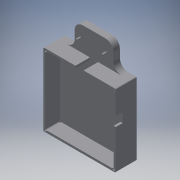
# Autodesk Inventor part: base
Saved by Autodesk Inventor 2019 (Build 230136000, 136)
## iProperties
Created: 2021-10-12
Part Number: base
Material: Generic
Document SubType Name: Modeling
Designer: Pulag
Density: 1 g/cm^3
Appearance: Default
Author: Pulag
Autodesk Inventor part; units mm, degrees
ref_plane "YZ Plane" through (0, 0, 0) normal (1, 0, 0) x (0, 1, 0)
ref_plane "XZ Plane" through (0, 0, 0) normal (0, 1, 0) x (-1, 0, 0)
ref_plane "XY Plane" through (0, 0, 0) normal (0, 0, 1) x (1, 0, 0)
sketch "Sketch1" plane through (0, 0, 0) normal (0, 0, 1) x (1, 0, 0)
  line L0 (-42.25, 42.25) -> (42.25, 42.25)
  line L1 (42.25, 42.25) -> (42.25, -42.25)
  line L2 (42.25, -42.25) -> (-42.25, -42.25)
  line L3 (-42.25, -42.25) -> (-42.25, 42.25)
  line L4 (-42.25, 42.25) -> (42.25, -42.25) construction
  line L5 (42.25, 42.25) -> (-42.25, -42.25) construction
  line L6 (-45, 45) -> (45, 45)
  line L7 (45, 45) -> (45, -45)
  line L8 (45, -45) -> (-45, -45)
  line L9 (-45, -45) -> (-45, 45)
  line L10 (-45, 45) -> (45, -45) construction
  line L11 (45, 45) -> (-45, -45) construction
  point P0 (0, 0)
  dimension "d0" = 84.5
  dimension "d1" = 84.5
  dimension "d2" = 90
  dimension "d3" = 90
  constraints: 24 end point, 4 midpoint, 4 parallel, 2 horizontal, 2 perpendicular
  measures "d0" distance of L1.end L2.end
  measures "d1" distance of L0.end L1.end
  measures "d2" distance of L7.end L8.end
  measures "d3" distance of L6.end L7.end
extrude "Extrusion1" add sketch "Sketch1" along normal blind 18
extrude "Extrusion2" add sketch "Sketch1" against normal blind 8 contours L0 L1 L2 L3 | L6 L7 L8 L9
sketch "Sketch2" plane through (0, 0, 18) normal (0, 0, 1) x (1, 0, 0)
  line L0 (42.25, -42.25) -> (42.25, 42.25) projected
  line L1 (42.25, 42.25) -> (-42.25, 42.25) projected
  line L2 (-42.25, 42.25) -> (-42.25, -42.25) projected
  line L3 (-42.25, -42.25) -> (42.25, -42.25) projected
  circle A0 centre (42.25, -42.25) radius 1.5
  line L4 (42.25, -42.25) -> (-42.25, -42.25) projected
  circle A1 centre (-42.25, -42.25) radius 1.5
  circle A2 centre (42.25, 42.25) radius 1.5
  line L5 (-42.25, 42.25) -> (42.25, 42.25) projected
  circle A3 centre (-42.25, 42.25) radius 1.5
  point P0 (0, 0)
  dimension "d8" = 3
  dimension "d9" = 3
  dimension "d10" = 3
  dimension "d11" = 3
  constraints: 4 centre point, 4 coincident
  measures "d8" diameter of A0
  measures "d9" diameter of A1
  measures "d10" diameter of A2
  measures "d11" diameter of A3
extrude "Extrusion3" cut sketch "Sketch2" against normal up to surface (18 mm away) contours L3 A0 L0 | L0 A0 L3 | A2 L1 L0 | L0 L1 A2 | A1 L2 L3 | L3 L2 A1 | A3 L2 L1 | L1 L2 A3
sketch "Sketch3" plane through (42.25, -40.75, 0) normal (-1, 0, 0) x (0, 0, 1)
  line L0 (18, 81.5) -> (0, 81.5) projected
  line L1 (0, 0) -> (0, 81.5) projected
  line L2 (0, 0) -> (18, 0) projected
  line L3 (18, 81.5) -> (18, 0) projected
  line L4 (9.5, 56.5) -> (19.5, 56.5)
  line L5 (19.5, 56.5) -> (19.5, 45)
  line L6 (19.5, 45) -> (9.5, 45)
  line L7 (9.5, 45) -> (9.5, 56.5)
  point P0 (0, 40.75)
  dimension "d14" = 10
  dimension "d15" = 11.5
  dimension "d16" = 25
  dimension "d17" = 9.5
  constraints: 8 end point, 2 parallel, 1 horizontal, 1 perpendicular
  measures "d14" distance of L5.end L6.end
  measures "d15" distance of L4.end L5.end
  measures "d16" distance between parallel lines of L4 L0
  measures "d17" distance between parallel lines of L1 L7
extrude "Extrusion4" cut sketch "Sketch3" against normal blind 10 contours L4 L5 L6 L3 | L3 L6 L7 L4
sketch "Sketch4" plane through (-40.75, 42.25, 0) normal (0, -1, 0) x (1, 0, 0)
  line L0 (0, 18) -> (0, 0) projected
  line L1 (81.5, 0) -> (0, 0) projected
  line L2 (81.5, 0) -> (81.5, 18) projected
  line L3 (0, 18) -> (81.5, 18) projected
  line L4 (0, 18) -> (81.5, 18) projected
  line L5 (81.5, 0) -> (0, 0) projected
  line L6 (45.75, 18) -> (35.75, 18)
  line L7 (35.75, 18) -> (35.75, 0)
  line L8 (35.75, 0) -> (45.75, 0)
  line L9 (45.75, 0) -> (45.75, 18)
  point P0 (40.75, 18)
  point P1 (40.75, 18)
  dimension "d22" = 10
  constraints: 8 end point, 2 midpoint, 2 parallel, 2 point on line, 1 coincident, 1 horizontal, 1 perpendicular
  measures "d22" distance of L8.end L7.end
extrude "Extrusion5" cut sketch "Sketch4" against normal up to surface (2.75 mm away) contours L3 L9 L1 L7
sketch "Sketch5" plane through (0, 0, -8) normal (0, 0, -1) x (-1, 0, 0)
  line L0 (45, 45) -> (-45, 45) projected
  line L1 (-45, 45) -> (-45, -45) projected
  line L2 (-45, -45) -> (45, -45) projected
  line L3 (45, -45) -> (45, 45) projected
  line L4 (-24, 45) -> (24, 45)
  line L5 (24, 45) -> (24, 75)
  line L6 (24, 75) -> (-24, 75)
  line L7 (-24, 75) -> (-24, 45)
  circle A0 centre (-15, 60) radius 1.3
  circle A1 centre (17, 60) radius 1.3
  point P0 (0, 0)
  point P1 (0, 45)
  point P2 (-24, 60)
  dimension "d25" = 48
  dimension "d26" = 30
  dimension "d27" = 2.6
  dimension "d28" = 2.6
  dimension "d29" = 32
  constraints: 8 end point, 3 midpoint, 2 centre point, 2 horizontal alignment, 2 parallel, 1 horizontal, 1 perpendicular
  measures "d25" distance of L6.end L5.end
  measures "d26" distance of L5.end L4.end
  measures "d27" diameter of A0
  measures "d28" diameter of A1
  measures "d29" distance of A1.centre A0.centre
extrude "Extrusion6" add sketch "Sketch5" against normal up to surface (8 mm away) contours L0 L7 L6 L5
extrude "Extrusion7" add sketch "Sketch5" against normal blind 5 from surface at -8 contours A0 | A1
fillet "Fillet1" radius 10 4 edges at (24, 75, -4) (-24, 75, -4) (24, 45, -4) (-24, 45, -4)
fillet "Fillet2" radius 1.5 4 edges at (45, 45, 5) (-45, 45, 5) (45, -45, 5) (-45, -45, 5)
sketch "Sketch6" plane through (0, 0, -8) normal (0, 0, -1) x (-1, 0, 0)
  circle A0 centre (18.3, -5) radius 6.1
  circle A1 centre (6.1, -5) radius 6.1
  circle A2 centre (-6.1, -5) radius 6.1
  circle A3 centre (-18.3, -5) radius 6.1
  line L0 (-43.5, -45) -> (43.5, -45) projected
  point P0 (0, 0)
  point P1 (0, -5)
  point P2 (0, -45)
  dimension "d38" = 12.2
  dimension "d39" = 12.2
  dimension "d37" = 12.2
  dimension "d40" = 12.2
  dimension "d41" = 40
  constraints: 5 horizontal alignment, 2 centre point, 1 midpoint, 1 vertical alignment, 6 other
  measures "d37" diameter of A0
  measures "d40" diameter of A3
  measures "d41" distance from line of L0 point (6.1, -5)
extrude "Extrusion8" cut sketch "Sketch6" against normal blind 1.6
body "Solid1"
